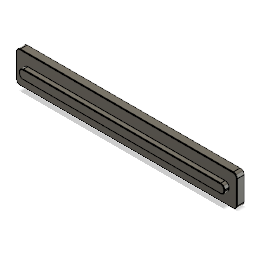
bed_extrusion_spacer_parametric (Autodesk Fusion 360 design; units mm, degrees)
Autodesk Fusion 360 part; units mm, degrees
sketch "Sketch1" plane through (0, 0, 0) normal (0, 0, 1) x (1, 0, 0)
  line L0 (0, 0) -> (140, 0)
  line L1 (140, 0) -> (140, 20)
  line L2 (140, 20) -> (0, 20)
  line L3 (0, 20) -> (0, 0)
  line L4 (5, 12.875) -> (135, 12.875)
  line L5 (135, 12.875) -> (135, 7.125)
  line L6 (135, 7.125) -> (5, 7.125)
  line L7 (5, 7.125) -> (5, 12.875)
  line L8 (70, 20) -> (70, 12.875) construction
  line L9 (70, 7.125) -> (70, 0) construction
  line L10 (70, 12.875) -> (70, 7.125) construction
  line L11 (0, 10) -> (5, 10) construction
  line L12 (140, 10) -> (135, 10) construction
  dimension "d1" = 140
  dimension "d2" = 5.75
  dimension "d3" = 20
  dimension "d11" = 5
  measures "d3" distance of L0.start
extrude "Extrude1" add sketch "Sketch1" against normal blind 5 contours L0 L1 L2 L3 | L4 L5 L6 L7
extrude "Extrude2" add sketch "Sketch1" along normal blind 3 contours L4 L5 L6 L7
fillet "Fillet1" radius 2.5 8 edges at (0, 0, -2.5) (0, 20, -2.5) (5, 7.125, 1.5) (5, 12.875, 1.5) (135, 12.875, 1.5) (135, 7.125, 1.5) (140, 20, -2.5) (140, 0, -2.5)
chamfer "Chamfer2" distance 0.3 angle 45 24 edges at (0, 10, -5) (0.7322, 0.7322, -5) (70, 0, -5) (139.2678, 0.7322, -5) (140, 10, -5) (139.2678, 19.2678, -5) (70, 20, -5) (0.7322, 19.2678, -5) (0.7322, 19.2678, 0) (0, 10, 0) (0.7322, 0.7322, 0) (70, 0, 0) (139.2678, 0.7322, 0) (140, 10, 0) (139.2678, 19.2678, 0) (70, 20, 0) (5.7322, 12.1428, 3) (5, 10, 3) (5.7322, 7.8572, 3) (70, 7.125, 3) (134.2678, 7.8572, 3) (135, 10, 3) (134.2678, 12.1428, 3) (70, 12.875, 3)
equation "d1 = SPACER_LENGTH"
equation "SPACER_LENGTH = 140 mm"
